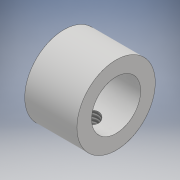
# Autodesk Inventor part: round_pd_holder_2
Saved by Autodesk Inventor 2017 (Build 210142000, 142)
## iProperties
Created: 2017-03-22
Part Number: round_pd_holder_2
Material: Generic
Document SubType Name: Modeling
Designer: Sam
Density: 1 g/cm^3
Appearance: Default
Author: Sam
Autodesk Inventor part; units mm, degrees
ref_plane "YZ Plane" through (0, 0, 0) normal (1, 0, 0) x (0, 1, 0)
ref_plane "XZ Plane" through (0, 0, 0) normal (0, 1, 0) x (-1, 0, 0)
ref_plane "XY Plane" through (0, 0, 0) normal (0, 0, 1) x (1, 0, 0)
sketch "Sketch1" plane through (0, 0, 0) normal (1, 0, 0) x (0, 1, 0)
  line L0 (0, 0) -> (15, 0)
  line L1 (15, 0) -> (15, -15)
  line L2 (15, -15) -> (0, -15)
  line L3 (0, -15) -> (0, 0)
  dimension "d0" = 15
  dimension "d1" = 15
  constraints: 8 end point, 2 parallel, 1 horizontal, 1 perpendicular
  measures "d0" distance of L1.end L2.end
  measures "d1" distance of L0.end L1.end
extrude "Extrusion1" add sketch "Sketch1" along normal blind 10
sketch "Sketch2" plane through (0, 0, -15) normal (0, 0, -1) x (-1, 0, 0)
  point P0 (0, 0)
  point P1 (-5, 7.5)
hole "Hole1" at (5, 7.5, -15) direction (0, 0, 1) diameter 3.242 depth 9.8 tip angle 118 thread size "M4x0.7" class "6H" standard "ANSI Metric M Profile"
sketch "Sketch3" plane through (10, 0, 0) normal (1, 0, 0) x (0, 0, -1)
  circle A0 centre (7.5, 7.5) radius 4.7
  point P0 (0, 0)
  dimension "d11" = 9.4
  constraints: 1 centre point
  measures "d11" diameter of A0
extrude "Extrusion2" cut sketch "Sketch3" against normal blind 10
fillet "Fillet1" radius 7.5 1 edges at (5, 15, -15)
fillet "Fillet2" radius 7.5 3 edges at (5, 0, -15) (5, 15, 0) (5, 0, 0)
body "Solid1"
